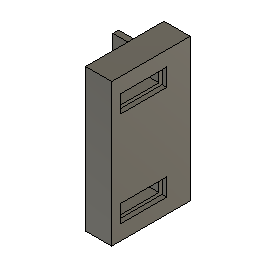
skadis_nut_right (Autodesk Fusion 360 design; units mm, degrees)
part number: 2026-09-06-14-40-23-923
Autodesk Fusion 360 part; units mm, degrees
sketch "Plate" plane through (0, 0, 0) normal (0, 1, 0) x (1, 0, 0)
  line L0 (0, 0) -> (11, 0)
  line L1 (11, 0) -> (11, -60)
  line L2 (11, -60) -> (0, -60)
  line L3 (0, -60) -> (0, 0)
  dimension "d36" = 11
  dimension "d37" = 60
  constraint coincident L0.start L3.end
  constraint horizontal L0
  constraint horizontal L2
  constraint vertical L1
  constraint vertical L3
  measures "d36" horizontal distance of L0.start L1.end
  measures "d37" vertical distance of L0.start L1.end
extrude "Plate (1)" add sketch "Plate" along normal mid plane 33 from surface at -4.5
sketch "Hook profile" plane through (0, 0, 0) normal (0, 1, 0) x (1, 0, 0)
  line L0 (0, -58) -> (-8.3, -58)
  line L1 (-8.3, -58) -> (-8.3, -41)
  line L2 (-8.3, -41) -> (-5.3, -41)
  line L3 (-5.3, -41) -> (-3.8, -42.5)
  line L4 (-3.8, -42.5) -> (-3.8, -53)
  line L5 (-3.8, -53) -> (0, -53)
  line L6 (0, -53) -> (0, -58)
  dimension "d41" = 58
  dimension "d42" = 8.3
  dimension "d43" = 3.8
  dimension "d44" = 5
  dimension "d45" = 10.5
  dimension "d46" = 1.5
  dimension "d47" = 1.5
  constraint horizontal L0
  constraint horizontal L2
  constraint horizontal L5
  constraint vertical L1
  constraint vertical L4
  constraint vertical L6
  constraint coincident origin L6
  measures "d41" vertical distance of origin L0.start
  measures "d42" horizontal distance of L0.start L0.end
  measures "d43" horizontal distance of L4.end L5.end
  measures "d44" vertical distance of L0.start L5.end
  measures "d45" vertical distance of L3.end L4.end
  measures "d46" horizontal distance of L2.end L3.end
  measures "d47" vertical distance of L2.end L3.end
extrude "Hook profile (1)" add sketch "Hook profile" along normal mid plane 2.4
pattern_linear "Hook rows" count 2 spacing 25.4 along (0, 0, -1) count 3 spacing 0 along (0, 0, 1) of "Hook profile (1)"
sketch "Nut channel" plane through (0, 0, 0) normal (0, 1, 0) x (1, 0, 0)
  line L0 (9, -46.3) -> (12, -46.3)
  line L1 (12, -46.3) -> (12, -53.7)
  line L2 (12, -53.7) -> (9, -53.7)
  line L3 (9, -53.7) -> (9, -46.3)
  dimension "d54" = 12
  dimension "d55" = 46.3
  dimension "d56" = 3
  dimension "d57" = 7.4
  constraint horizontal L0
  constraint horizontal L2
  constraint vertical L1
  constraint vertical L3
  measures "d54" horizontal distance of origin L0.end
  measures "d55" vertical distance of origin L0.end
  measures "d56" horizontal distance of L0.start L0.end
  measures "d57" vertical distance of L0.end L1.end
extrude "Nut channel (1)" cut sketch "Nut channel" along normal mid plane 19.4 from surface at -7.52
pattern_linear "Nut channel rows" count 2 spacing 40 along (0, 0, -1) count 3 spacing 0 along (0, 0, 1) of "Nut channel (1)"
sketch "Screw relief" plane through (0, 0, 0) normal (0, 1, 0) x (1, 0, 0)
  line L0 (-1, -47.6) -> (12, -47.6)
  line L1 (12, -47.6) -> (12, -52.4)
  line L2 (12, -52.4) -> (-1, -52.4)
  line L3 (-1, -52.4) -> (-1, -47.6)
  dimension "d65" = 12
  dimension "d66" = 47.6
  dimension "d67" = 13
  dimension "d68" = 4.8
  constraint horizontal L0
  constraint horizontal L2
  constraint vertical L1
  constraint vertical L3
  measures "d65" horizontal distance of origin L0.end
  measures "d66" vertical distance of origin L0.end
  measures "d67" horizontal distance of L0.start L0.end
  measures "d68" vertical distance of L0.end L1.end
extrude "Screw relief (1)" cut sketch "Screw relief" along normal mid plane 16.8 from surface at -7.52
pattern_linear "Screw relief rows" count 2 spacing 40 along (0, 0, -1) count 3 spacing 0 along (0, 0, 1) of "Screw relief (1)"
equation "bracketWidth = 24.0 mm" comment "bracket width across the upright"
equation "plateHeight = 60.0 mm" comment "plate height"
equation "plateInboardExtension = 9.0 mm" comment "extra plate toward the desk centre, where the channel reaches"
equation "boardThickness = 6.0 mm" comment "measured SKADIS panel thickness"
equation "screwLength = 15.0 mm" comment "measured decorative M4 screw"
equation "screwDiameter = 4.0 mm" comment "M4 shank"
equation "screwClearance = 0.8 mm" comment "slack around the shank"
equation "screwTipClearance = 2.2 mm" comment "tip stops this short of the plate's back face"
equation "screwSlotWidth = screwDiameter + screwClearance" comment "screw relief slot height"
equation "nutAcrossFlats = 7.0 mm" comment "M4 square nut across flats"
equation "nutThickness = 2.2 mm" comment "M4 square nut thickness"
equation "nutChannelClearance = 0.4 mm" comment "slack around the nut in its channel"
equation "nutProud = 0.2 mm" comment "nut stands out of the pocket to be clamped"
equation "nutPocketDepth = nutThickness - nutProud" comment "channel depth"
equation "nutChannelHeight = nutAcrossFlats + nutChannelClearance" comment "channel height; under the nut's diagonal so it cannot turn"
equation "plateThickness = screwLength - boardThickness - nutProud + screwTipClearance" comment "derived: deep enough to swallow the screw"
equation "mountTravel = 12.0 mm" comment "left-right adjustment"
equation "nutChannelLength = mountTravel + nutAcrossFlats + nutChannelClearance" comment "channel length along the plate"
equation "screwSlotLength = mountTravel + screwSlotWidth" comment "relief slot length along the plate"
equation "topMountZ = 50.0 mm" comment "top channel centre"
equation "mountOffsetY = -7.52 mm" comment "channel centre on the board's grid"
equation "slotOvershoot = 1.0 mm" comment "cuts reach past the faces they cut"
equation "slotWidth = 3.2 mm" comment "measured upright slot width"
equation "slotPitchVertical = 25.4 mm" comment "1 inch, measured"
equation "faceMetalThickness = 2.0 mm" comment "upright face metal"
equation "hookTabWidth = slotWidth - 0.8 mm" comment "blade width through the slot"
equation "hookThroat = faceMetalThickness + 1.8 mm" comment "gap behind the plate"
equation "hookNeckHeight = 5.0 mm" comment "bears on the slot bottom edge"
equation "hookLipThickness = 4.5 mm" comment "lip behind the upright face"
equation "hookLipDrop = 12.0 mm" comment "engagement below the neck"
equation "hookLipChamfer = 1.5 mm" comment "lead-in past slot burrs"
equation "topHookNeckTop = plateHeight - 2 mm" comment "top hook row"
equation "hookRows = 2" comment "hook rows (pattern count)"
equation "boardPitch = 40.0 mm" comment "SKADIS grid pitch"
equation "mountRows = 2" comment "channels per bracket (pattern count)"
equation "d36 = plateThickness"
equation "d37 = plateHeight"
equation "d38 = -plateInboardExtension / 2"
equation "d39 = bracketWidth + plateInboardExtension"
equation "d41 = topHookNeckTop"
equation "d42 = hookThroat + hookLipThickness"
equation "d43 = hookThroat"
equation "d44 = hookNeckHeight"
equation "d45 = hookLipDrop - hookLipChamfer"
equation "d46 = hookLipChamfer"
equation "d47 = hookLipChamfer"
equation "d48 = hookTabWidth"
equation "d50 = hookRows"
equation "d52 = -slotPitchVertical"
equation "d54 = plateThickness + slotOvershoot"
equation "d55 = topMountZ - nutChannelHeight / 2"
equation "d56 = nutPocketDepth + slotOvershoot"
equation "d57 = nutChannelHeight"
equation "d58 = mountOffsetY"
equation "d59 = nutChannelLength"
equation "d61 = mountRows"
equation "d63 = -boardPitch"
equation "d65 = plateThickness + slotOvershoot"
equation "d66 = topMountZ - screwSlotWidth / 2"
equation "d67 = plateThickness + 2 * slotOvershoot"
equation "d68 = screwSlotWidth"
equation "d69 = mountOffsetY"
equation "d70 = screwSlotLength"
equation "d72 = mountRows"
equation "d74 = -boardPitch"
named bodies: "skadis_nut_right"
